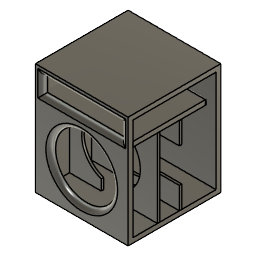
Sub Woofer Enclosure (Autodesk Fusion 360 design; units mm, degrees)
part number: 2026-03-23-19-17-00-272
Autodesk Fusion 360 part; units mm, degrees
sketch "Sketch1" plane through (0, 0, 0) normal (0, 0, 1) x (1, 0, 0)
  line L0 (-190, 190) -> (190, 190)
  line L1 (190, 190) -> (190, -190)
  line L2 (190, -190) -> (-190, -190)
  line L3 (-190, -190) -> (-190, 190)
  dimension "d1" = 380
  dimension "d2" = 380
  dimension "d3" = 190
  dimension "d4" = 190
  constraint horizontal L0
  constraint vertical L1
  constraint horizontal L2
  constraint vertical L3
  measures "d1" distance of L0.start L0.end
  measures "d2" distance of L0.start L2.end
  measures "d3" distance of origin L0
  measures "d4" distance of origin L3
extrude "Extrude1" add sketch "Sketch1" along normal blind 457 makes body 1
shell "Shell1" thickness 20 removed faces 1 at (190, 63.3333, 152.3333) on bodies 1
hole "Hole1" at (0.0793, -190, 176.2155) direction (0, 1, 0) diameter 254 depth 100 tip angle 180 bodies 1
fillet "Fillet1" radius 20 1 edges at (46.0044, -190, 294.6211) on bodies 1
sketch "Sketch2" plane through (0, -190, 0) normal (0, -1, 0) x (1, 0, 0)
  line L0 (-190, 0) -> (190, 0)
  line L1 (190, 0) -> (190, 457)
  line L2 (190, 457) -> (-190, 457)
  line L3 (-190, 457) -> (-190, 0)
  circle A0 centre (0.0793, 176.2155) radius 147
  line L4 (-160, 425) -> (160, 425)
  line L5 (160, 425) -> (160, 360)
  line L6 (160, 360) -> (-160, 360)
  line L7 (-160, 360) -> (-160, 425)
  constraint horizontal L4
  constraint vertical L5
  constraint horizontal L6
  constraint vertical L7
extrude "Extrude2" cut sketch "Sketch2" against normal blind 50 contours L4 L5 L6 L7 bodies 1
fillet "Fillet2" radius 20 4 edges at (0, -190, 425) (-160, -190, 392.5) (0, -190, 360) (160, -190, 392.5) on bodies 1
sketch "Sketch4" plane through (0, 0, 0) normal (0, 0, 1) x (1, 0, 0)
  line L0 (-190, -190) -> (190, -190)
  line L1 (190, -190) -> (190, 117.5)
  line L2 (190, 117.5) -> (-190, 117.5)
  line L3 (-190, 117.5) -> (-190, -190)
  constraint horizontal L0
  constraint vertical L1
  constraint horizontal L2
  constraint vertical L3
extrude "Extrude3" add sketch "Sketch4" along normal blind 20 separate body makes body 2
move_body "Move1" bodies 2 to x (1, 0, 0) y (0, 1, 0) z (0, 0, 1) at (0, 0, 340)
move_body "Move2" bodies 2 to x (1, 0, 0) y (0, 1, 0) z (0, 0, 1) at (-1, 20, 0)
fillet "Fillet3" radius 10 1 faces at (62.3333, 137.5, 346.6667) on bodies 2
sketch "Sketch5" plane through (0, 170, 0) normal (0, -1, 0) x (1, 0, 0)
  circle A0 centre (0.0793, 176.2155) radius 147
  line L0 (-190, 0) -> (190, 0)
  line L1 (190, 0) -> (190, 457)
  line L2 (190, 457) -> (-190, 457)
  line L3 (-190, 457) -> (-190, 0)
  line L4 (180, 445) -> (180, 340)
  line L5 (180, 340) -> (-180, 340)
  line L6 (-180, 340) -> (-180, 445)
  line L7 (-180, 445) -> (180, 445)
  circle A1 centre (0.0793, 176.2155) radius 120
  line L8 (-190, 0) -> (-40, 0)
  line L9 (-40, 0) -> (-40, 340)
  line L10 (-40, 340) -> (-190, 340)
  line L11 (-190, 340) -> (-190, 0)
  line L12 (190, 0) -> (40, 0)
  line L13 (40, 0) -> (40, 340)
  line L14 (40, 340) -> (190, 340)
  line L15 (190, 340) -> (190, 0)
  line L16 (-170, 20) -> (190, 20)
  line L17 (190, 20) -> (190, 437)
  line L18 (190, 437) -> (-170, 437)
  line L19 (-170, 437) -> (-170, 20)
  line L20 (-190, 340) -> (190, 340)
  line L21 (190, 340) -> (190, 250)
  line L22 (190, 250) -> (-190, 250)
  line L23 (-190, 250) -> (-190, 340)
  line L24 (-190, 0) -> (190, 0)
  line L25 (190, 0) -> (190, 110)
  line L26 (190, 110) -> (-190, 110)
  line L27 (-190, 110) -> (-190, 0)
  dimension "d21" = 240
  constraint coincident A0.centre A1.centre
  constraint horizontal L8
  constraint vertical L9
  constraint horizontal L10
  constraint vertical L11
  constraint coincident L5 L9.end
  constraint coincident L0.start L3.end
  constraint horizontal L12
  constraint vertical L13
  constraint horizontal L14
  constraint vertical L15
  constraint coincident L5 L13.end
  constraint coincident L0.end L1.start
  constraint horizontal L20
  constraint vertical L21
  constraint horizontal L22
  constraint vertical L23
  constraint coincident L15 L21.end
  constraint horizontal L24
  constraint vertical L25
  constraint horizontal L26
  constraint vertical L27
  constraint coincident L15 L25.end
  measures "d21" diameter of A1
extrude "Extrude5" add sketch "Sketch5" along normal blind 10 from surface at 230 separate body contours A0 A1 L22 L26 | A0 L1 L15 L17 L22 L26 | A0 A1 L13 L22 | A0 L1 L5 L13 L14 L15 L17 L20 L21 L22 | A0 L1 L13 L15 L16 L17 L25 L26 | A0 A1 L13 L26 | A0 A1 L9 L22 | A0 L5 L9 L10 L19 L20 L22 | A0 L9 L16 L19 L26 | A0 A1 L9 L26 | A0 A1 L22 L26 | A0 L19 L22 L26 makes body 3 at (166.5881, -60, 181.634) makes body 4 at (-93.5397, -60, 317.726)
extrude "Extrude6" add sketch "Sketch5" along normal blind 10 from surface at 140 separate body contours A0 A1 L13 L22 | A0 L1 L5 L13 L14 L15 L17 L20 L21 L22 | A0 L1 L13 L15 L16 L17 L25 L26 | A0 A1 L13 L26 | A0 A1 L9 L13 | A0 L5 L9 L13 L20 | A0 L9 L13 L16 | A0 A1 L9 L13 | A0 A1 L9 L22 | A0 L5 L9 L10 L19 L20 L22 | A0 L9 L16 L19 L26 | A0 A1 L9 L26 makes body 5 at (158.2382, 20, 280) makes body 6 at (160.0522, 20, 80)
